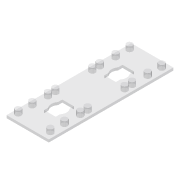
# Autodesk Inventor part: 00_FluidicChip_AlexSwen
Saved by Autodesk Inventor 2019 (Build 230136000, 136)
## iProperties
Created: 2019-07-01
Part Number: 00_FluidicChip_AlexSwen
Material: Generic
Document SubType Name: Modeling
Designer: diederichbenedict
Density: 1 g/cm^3
Appearance: Polycarbonate - Clear
Author: diederichbenedict
Autodesk Inventor part; units mm, degrees
ref_plane "YZ Plane" through (0, 0, 0) normal (1, 0, 0) x (0, 1, 0)
ref_plane "XZ Plane" through (0, 0, 0) normal (0, 1, 0) x (-1, 0, 0)
ref_plane "XY Plane" through (0, 0, 0) normal (0, 0, 1) x (1, 0, 0)
sketch "Sketch1" plane through (0, 0, 0) normal (0, 1, 0) x (-1, 0, 0)
  line L0 (0, 0) -> (25.5, 0)
  line L1 (25.5, 0) -> (25.5, -75.4)
  line L2 (25.5, -75.4) -> (0, -75.4)
  line L3 (0, -75.4) -> (0, 0)
  dimension "d0" = 25.5
  dimension "d1" = 75.4
  constraints: 8 end point, 2 parallel, 1 horizontal, 1 perpendicular
  measures "d0" distance of L1.end L2.end
  measures "d1" distance of L0.end L1.end
extrude "Extrusion1" add sketch "Sketch1" along normal blind 1.6
sketch "Sketch2" plane through (0, 1.6, 0) normal (0, 1, 0) x (1, 0, 0)
  line L0 (-25.5, 0) -> (0, 0) projected
  line L1 (0, 0) -> (0, 75.4) projected
  line L2 (0, 75.4) -> (-25.5, 75.4) projected
  line L3 (-25.5, 75.4) -> (-25.5, 0) projected
  circle A0 centre (-22.5, 71.4) radius 1.75
  circle A1 centre (-22.5, 62.9) radius 1.75
  circle A2 centre (-22.5, 53.4) radius 1.75
  circle A3 centre (-22.5, 48.9) radius 1.75
  line L4 (-25.5, 0) -> (0, 0) construction
  line L5 (-12.75, 0) -> (-12.75, 75.4) construction
  line L6 (0, 75.4) -> (-25.5, 75.4) construction
  line L7 (-25.5, 75.4) -> (-25.5, 0) construction
  line L8 (-25.5, 37.7) -> (0, 37.7) construction
  circle A4 centre (-3, 71.4) radius 1.75
  circle A5 centre (-3, 62.9) radius 1.75
  circle A6 centre (-3, 53.4) radius 1.75
  circle A7 centre (-3, 48.9) radius 1.75
  circle A8 centre (-22.5, 4) radius 1.75
  circle A9 centre (-22.5, 12.5) radius 1.75
  circle A10 centre (-22.5, 22) radius 1.75
  circle A11 centre (-22.5, 26.5) radius 1.75
  circle A12 centre (-3, 22) radius 1.75
  circle A13 centre (-3, 12.5) radius 1.75
  circle A14 centre (-3, 4) radius 1.75
  circle A15 centre (-3, 26.5) radius 1.75
  dimension "d4" = 3.5
  dimension "d5" = 3
  dimension "d6" = 4
  dimension "d7" = 3.5
  dimension "d8" = 12.5
  dimension "d9" = 3.5
  dimension "d10" = 22
  dimension "d11" = 3.5
  dimension "d12" = 26.5
  constraints: 16 centre point, 12 symmetric about line, 4 end point, 4 midpoint, 12 other
  measures "d4" diameter of A0
  measures "d5" distance from line of A0.centre L3
  measures "d6" distance from line of A0.centre L2
  measures "d7" diameter of A1
  measures "d8" distance from line of L2 A1.centre
  measures "d9" diameter of A2
  measures "d10" distance from line of L2 A2.centre
  measures "d11" diameter of A3
  measures "d12" distance from line of A3.centre L2
extrude "Extrusion2" add sketch "Sketch2" along normal blind 3 contours A0 | A1 | A2 | A3 | A4 | A5 | A6 | A7 | A8 | A9 | A10 | A11 | A12 | A13 | A14 | A15
sketch "Sketch3" plane through (0, 1.6, 0) normal (0, 1, 0) x (1, 0, 0)
  circle A0 centre (-22.5, 4) radius 1.75 projected
  circle A1 centre (-22.5, 12.5) radius 1.75 projected
  circle A2 centre (-22.5, 22) radius 1.75 projected
  circle A3 centre (-22.5, 26.5) radius 1.75 projected
  circle A4 centre (-3, 71.4) radius 1.75 projected
  circle A5 centre (-3, 53.4) radius 1.75 projected
  circle A6 centre (-22.5, 53.4) radius 1.75 projected
  circle A7 centre (-22.5, 71.4) radius 1.75 projected
  circle A8 centre (-22.5, 62.9) radius 1.75 projected
  circle A9 centre (-22.5, 48.9) radius 1.75 projected
  circle A10 centre (-3, 62.9) radius 1.75 projected
  circle A11 centre (-3, 48.9) radius 1.75 projected
  circle A12 centre (-3, 26.5) radius 1.75 projected
  circle A13 centre (-3, 22) radius 1.75 projected
  circle A14 centre (-3, 12.5) radius 1.75 projected
  circle A15 centre (-3, 4) radius 1.75 projected
  line L0 (-25.5, 0) -> (0, 0) projected
  line L1 (0, 0) -> (0, 75.4) projected
  line L2 (0, 75.4) -> (-25.5, 75.4) projected
  line L3 (-25.5, 75.4) -> (-25.5, 0) projected
  line L4 (-16.8, 61.4) -> (-9.8, 61.4)
  line L5 (-9.8, 61.4) -> (-9.8, 50.4)
  line L6 (-9.8, 50.4) -> (-16.8, 50.4)
  line L7 (-16.8, 50.4) -> (-16.8, 61.4)
  line L8 (-25.5, 0) -> (-25.5, 75.4) projected
  line L9 (-25.5, 37.7) -> (0, 37.7)
  line L10 (0, 75.4) -> (0, 0) projected
  line L11 (-16.8, 14) -> (-9.8, 14)
  line L12 (-9.8, 14) -> (-9.8, 25)
  line L13 (-9.8, 25) -> (-16.8, 25)
  line L14 (-16.8, 25) -> (-16.8, 14)
  circle A16 centre (-13.3, 55.9) radius 4.511
  circle A17 centre (-13.3, 19.5) radius 4.5729
  dimension "d15" = 7
  dimension "d16" = 11
  dimension "d17" = 14
  dimension "d18" = 8.7
  constraints: 18 end point, 4 symmetric about line, 2 centre point, 2 midpoint, 2 parallel, 1 horizontal, 1 perpendicular
  measures "d15" distance of L5.end L6.end
  measures "d16" distance of L4.end L5.end
  measures "d17" distance between parallel lines of L4 L2
  measures "d18" distance between parallel lines of L7 L3
extrude "Extrusion3" cut sketch "Sketch3" against normal blind 3 contours L4 L5 A16 L7 | A16 L5 L7 | L7 A16 | A16 L5 | A16 L5 L6 L7 | L14 A17 L12 L11 | A17 L14 | L14 A17 L12 | L12 A17 | L14 L13 L12 A17
body "Solid1"
